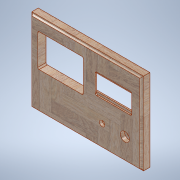
# Autodesk Inventor part: EW_Holzplatte
Saved by Autodesk Inventor 2020 (Build 240168000, 168)
## iProperties
Created: 2020-06-21
Part Number: EW_Holzplatte
Material: Eiche, Rot
Document SubType Name: Modeling
Designer: Johannes
Density: 0.673 g/cm^3
Appearance: Eiche - Fischgrätmuster
Author: Johannes
Autodesk Inventor part; units mm, degrees
ref_plane "YZ Plane" through (0, 0, 0) normal (1, 0, 0) x (0, 1, 0)
ref_plane "XZ Plane" through (0, 0, 0) normal (0, 1, 0) x (-1, 0, 0)
ref_plane "XY Plane" through (0, 0, 0) normal (0, 0, 1) x (1, 0, 0)
sketch "Skizze1" plane through (0, 0, 0) normal (0, 0, 1) x (1, 0, 0)
  line L0 (-122.5, 90) -> (122.5, 90)
  line L1 (122.5, 90) -> (122.5, -90)
  line L2 (122.5, -90) -> (-122.5, -90)
  line L3 (-122.5, -90) -> (-122.5, 90)
  line L4 (-122.5, 90) -> (122.5, -90) construction
  line L5 (122.5, 90) -> (-122.5, -90) construction
  point P0 (0, 0)
  dimension "d0" = 245
  dimension "d1" = 180
  constraints: 12 end point, 2 midpoint, 2 parallel, 1 horizontal, 1 perpendicular
  measures "d0" distance of L1.end L2.end
  measures "d1" distance of L0.end L1.end
extrude "Extrusion1" add sketch "Skizze1" along normal blind 18
sketch "Skizze3" plane through (0, 0, 18) normal (0, 0, 1) x (1, 0, 0)
  line L0 (20.5, 50.5) -> (100.5, 50.5)
  line L1 (100.5, 50.5) -> (100.5, 5.5)
  line L2 (100.5, 5.5) -> (20.5, 5.5)
  line L3 (20.5, 5.5) -> (20.5, 50.5)
  line L4 (20.5, 50.5) -> (100.5, 5.5) construction
  line L5 (100.5, 50.5) -> (20.5, 5.5) construction
  line L6 (122.5, 90) -> (-122.5, 90) projected
  line L7 (122.5, -90) -> (122.5, 90) projected
  point P0 (0, 0)
  point P1 (60.5, 28)
  dimension "d12" = 80
  dimension "d13" = 45
  dimension "d32" = 62
  dimension "d33" = 62
  constraints: 12 end point, 2 midpoint, 2 parallel, 1 horizontal, 1 perpendicular
  measures "d12" distance of L0.start L0.end
  measures "d13" distance of L2.end L0.start
  measures "d32" distance from line of L6 point (60.5, 28)
  measures "d33" distance from line of L7 point (60.5, 28)
extrude "Extrusion2" cut sketch "Skizze3" against normal blind 3
sketch "Skizze4" plane through (0, 0, 0) normal (0, 0, -1) x (-1, 0, 0)
  line L0 (-113, 69.75) -> (-8, 69.75)
  line L1 (-8, 69.75) -> (-8, -27.25)
  line L2 (-8, -27.25) -> (-113, -27.25)
  line L3 (-113, -27.25) -> (-113, 69.75)
  line L4 (-113, 69.75) -> (-8, -27.25) construction
  line L5 (-8, 69.75) -> (-113, -27.25) construction
  line L6 (-122.5, 90) -> (122.5, 90) projected
  line L7 (-122.5, -90) -> (-122.5, 90) projected
  point P0 (0, 0)
  point P1 (-60.5, 21.25)
  dimension "d20" = 62
  dimension "d21" = 105
  dimension "d22" = 97
  dimension "d23" = 20.25
  constraints: 12 end point, 2 midpoint, 2 parallel, 1 horizontal, 1 perpendicular
  measures "d20" distance from line of L7 point (-60.5, 21.25)
  measures "d21" distance of L0.start L0.end
  measures "d22" distance of L2.end L0.start
  measures "d23" distance between parallel lines of L0 L6
extrude "Extrusion3" cut sketch "Skizze4" against normal blind 6
sketch "Skizze5" plane through (0, 0, 6) normal (0, 0, -1) x (-1, 0, 0)
  line L0 (-113, 49) -> (-8, 49)
  line L1 (-8, 49) -> (-8, -6)
  line L2 (-8, -6) -> (-113, -6)
  line L3 (-113, -6) -> (-113, 49)
  line L4 (-113, 49) -> (-8, -6) construction
  line L5 (-8, 49) -> (-113, -6) construction
  line L6 (-122.5, 90) -> (122.5, 90) projected
  line L7 (-122.5, -90) -> (-122.5, 90) projected
  point P0 (0, 0)
  point P1 (-60.5, 21.5)
  dimension "d26" = 105
  dimension "d34" = 62
  dimension "d35" = 41
  dimension "d36" = 96
  constraints: 12 end point, 2 midpoint, 2 parallel, 1 horizontal, 1 perpendicular
  measures "d26" distance of L0.start L0.end
  measures "d34" distance from line of L7 point (-60.5, 21.5)
  measures "d35" distance between parallel lines of L6 L0
  measures "d36" distance between parallel lines of L2 L6
extrude "Extrusion4" cut sketch "Skizze5" against normal blind 6
sketch "Skizze14" plane through (0, 0, 12) normal (0, 0, -1) x (-1, 0, 0)
  line L0 (-113, 45.5) -> (-8, 45.5)
  line L1 (-8, 45.5) -> (-8, 10.5)
  line L2 (-8, 10.5) -> (-113, 10.5)
  line L3 (-113, 10.5) -> (-113, 45.5)
  line L4 (-113, 45.5) -> (-8, 10.5) construction
  line L5 (-8, 45.5) -> (-113, 10.5) construction
  line L6 (-122.5, -90) -> (-122.5, 90) projected
  line L7 (-122.5, 90) -> (122.5, 90) projected
  line L8 (-113, -27.25) -> (-113, 69.75) projected
  point P0 (0, 0)
  point P1 (-60.5, 28)
  dimension "d72" = 62
  dimension "d73" = 62
  dimension "d74" = 35
  constraints: 12 end point, 2 midpoint, 2 parallel, 1 collinear, 1 horizontal, 1 perpendicular
  measures "d72" distance from line of L6 point (-60.5, 28)
  measures "d73" distance from line of L7 point (-60.5, 28)
  measures "d74" distance of L2.end L0.start
extrude "Extrusion11" cut sketch "Skizze14" against normal blind 3
sketch "Skizze7" plane through (0, 0, 0) normal (0, 0, -1) x (-1, 0, 0)
  circle A0 centre (-35.5, -41.5) radius 6
  circle A1 centre (-85.5, -41.5) radius 3.5
  line L0 (-122.5, -90) -> (-122.5, 90) projected
  line L1 (-122.5, 90) -> (122.5, 90) projected
  point P0 (0, 0)
  dimension "d44" = 37
  dimension "d45" = 50
  dimension "d46" = 12
  dimension "d47" = 7
  dimension "d48" = 131.5
  constraints: 2 centre point, 1 horizontal alignment
  measures "d44" distance from line of L0 A1.centre
  measures "d45" distance of A0.centre A1.centre
  measures "d46" diameter of A0
  measures "d47" diameter of A1
  measures "d48" distance from line of L1 A0.centre
extrude "Extrusion6" cut sketch "Skizze7" against normal through all
sketch "Skizze8" plane through (0, 0, 0) normal (0, 0, -1) x (-1, 0, 0)
  line L0 (-43.5, -23.5) -> (-27.5, -23.5)
  line L1 (-27.5, -23.5) -> (-27.5, -59.5)
  line L2 (-27.5, -59.5) -> (-43.5, -59.5)
  line L3 (-43.5, -59.5) -> (-43.5, -23.5)
  line L4 (-43.5, -23.5) -> (-27.5, -59.5) construction
  line L5 (-27.5, -23.5) -> (-43.5, -59.5) construction
  circle A0 centre (-35.5, -41.5) radius 6 projected
  point P0 (0, 0)
  point P1 (-35.5, -41.5)
  dimension "d51" = 16
  dimension "d52" = 36
  constraints: 12 end point, 3 midpoint, 2 parallel, 1 coincident, 1 horizontal, 1 perpendicular
  measures "d51" distance of L0.start L0.end
  measures "d52" distance of L0.end L1.end
extrude "Extrusion7" cut sketch "Skizze8" against normal blind 12
sketch "Skizze9" plane through (0, 0, 0) normal (0, 0, -1) x (-1, 0, 0)
  line L0 (-91.5, -30.5) -> (-79.5, -30.5)
  line L1 (-79.5, -30.5) -> (-79.5, -52.5)
  line L2 (-79.5, -52.5) -> (-91.5, -52.5)
  line L3 (-91.5, -52.5) -> (-91.5, -30.5)
  circle A0 centre (-85.5, -41.5) radius 3.5 projected
  line L4 (-91.5, -30.5) -> (-79.5, -52.5) construction
  line L5 (-79.5, -30.5) -> (-91.5, -52.5) construction
  point P0 (0, 0)
  dimension "d55" = 12
  dimension "d56" = 22
  constraints: 12 end point, 2 midpoint, 2 parallel, 1 horizontal, 1 perpendicular
  measures "d55" distance of L1.end L2.end
  measures "d56" distance of L0.end L1.end
extrude "Extrusion8" cut sketch "Skizze9" against normal blind 5
sketch "Skizze10" plane through (0, 0, 18) normal (0, 0, 1) x (1, 0, 0)
  circle A0 centre (85.5, -41.5) radius 3.5 projected
  circle A1 centre (85.5, -41.5) radius 10
  point P0 (0, 0)
  dimension "d59" = 20
  constraints: 1 centre point, 1 coincident
  measures "d59" diameter of A1
extrude "Extrusion9" cut sketch "Skizze10" against normal blind 9
sketch "Skizze11" plane through (0, 0, 0) normal (0, 0, -1) x (-1, 0, 0)
  line L0 (5.5, 64) -> (105.5, 64)
  line L1 (105.5, 64) -> (105.5, -8)
  line L2 (105.5, -8) -> (5.5, -8)
  line L3 (5.5, -8) -> (5.5, 64)
  line L4 (5.5, 64) -> (105.5, -8) construction
  line L5 (105.5, 64) -> (5.5, -8) construction
  line L6 (-122.5, 90) -> (122.5, 90) projected
  line L7 (122.5, 90) -> (122.5, -90) projected
  point P0 (0, 0)
  point P1 (55.5, 28)
  dimension "d62" = 26
  dimension "d63" = 17
  dimension "d64" = 100
  dimension "d65" = 72
  constraints: 12 end point, 2 midpoint, 2 parallel, 1 horizontal, 1 perpendicular
  measures "d62" distance between parallel lines of L6 L0
  measures "d63" distance between parallel lines of L7 L1
  measures "d64" distance of L0.start L0.end
  measures "d65" distance of L0.end L1.end
extrude "Extrusion10" cut sketch "Skizze11" against normal through all
sketch "Skizze15" plane through (0, 0, 0) normal (0, 0, -1) x (-1, 0, 0)
  line L0 (105.5, -8) -> (5.5, -8) projected
  line L1 (5.5, -8) -> (-11, -8)
  line L2 (-11, -8) -> (-11, 49)
  line L3 (-11, 49) -> (5.5, 49)
  line L4 (5.5, 49) -> (5.5, -8)
  line L5 (-8, 69.75) -> (-8, -27.25) projected
  line L6 (-113, 49) -> (-8, 49) projected
  point P0 (0, 0)
  dimension "d80" = 3
  constraints: 8 end point, 2 parallel, 1 horizontal, 1 perpendicular, 1 point on line, 1 other
extrude "Extrusion12" cut sketch "Skizze15" against normal up to surface (12 mm away)
fillet "Rundung1" radius 3 32 edges at (20.5, 50.5, 16.5) (20.5, 5.5, 16.5) (100.5, 5.5, 16.5) (100.5, 50.5, 16.5) (113, 69.75, 3) (8, 69.75, 3) (8, -27.25, 3) (113, -27.25, 3) (113, 49, 9) (8, 49, 3) (113, -6, 9) (43.5, -27.25, 3) (27.5, -27.25, 3) (27.5, -23.5, 9) (43.5, -23.5, 9) (43.5, -59.5, 6) (27.5, -59.5, 6) (91.5, -30.5, 2.5) (79.5, -30.5, 2.5) (79.5, -52.5, 2.5) (91.5, -52.5, 2.5) (-5.5, 64, 9) (-5.5, -8, 15) (-105.5, -8, 9) (-105.5, 64, 9) (113, 45.5, 13.5) (113, 10.5, 13.5) (8, 45.5, 13.5) (8, 10.5, 13.5) (8, -8, 3) (-5.5, 49, 6) (11, -8, 9)
sketch "Skizze12" plane through (0, 0, 0) normal (1, 0, 0) x (0, 1, 0)
  circle A0 centre (90, 18) radius 4
  point P0 (0, 0)
  dimension "d69" = 8
  constraints: 1 centre point, 1 coincident
  measures "d69" diameter of A0
sketch "Skizze13" plane through (0, 0, 18) normal (0, 0, 1) x (1, 0, 0)
  line L0 (-122.5, 90) -> (-122.5, -90) projected
  line L1 (-122.5, -90) -> (122.5, -90) projected
  line L2 (122.5, -90) -> (122.5, 90) projected
  line L3 (122.5, 90) -> (-122.5, 90) projected
  line L4 (-102.5, 64) -> (-8.5, 64) projected
  arc A0 (-5.5, 61) -> (-8.5, 64) centre (-8.5, 61) ccw projected
  line L5 (-5.5, 61) -> (-5.5, -5) projected
  arc A1 (-8.5, -8) -> (-5.5, -5) centre (-8.5, -5) ccw projected
  line L6 (-8.5, -8) -> (-102.5, -8) projected
  arc A2 (-105.5, -5) -> (-102.5, -8) centre (-102.5, -5) ccw projected
  line L7 (-105.5, -5) -> (-105.5, 61) projected
  arc A3 (-102.5, 64) -> (-105.5, 61) centre (-102.5, 61) ccw projected
  circle A4 centre (85.5, -41.5) radius 10 projected
  circle A5 centre (35.5, -41.5) radius 6 projected
  line L8 (20.5, 8.5) -> (20.5, 47.5) projected
  arc A6 (23.5, 50.5) -> (20.5, 47.5) centre (23.5, 47.5) ccw projected
  line L9 (23.5, 50.5) -> (97.5, 50.5) projected
  arc A7 (100.5, 47.5) -> (97.5, 50.5) centre (97.5, 47.5) ccw projected
  line L10 (100.5, 47.5) -> (100.5, 8.5) projected
  arc A8 (97.5, 5.5) -> (100.5, 8.5) centre (97.5, 8.5) ccw projected
  line L11 (97.5, 5.5) -> (23.5, 5.5) projected
  arc A9 (20.5, 8.5) -> (23.5, 5.5) centre (23.5, 8.5) ccw projected
  point P0 (0, 0)
sweep "Sweeping1" cut profiles "Skizze12" path "Skizze13" path curves L1 L0 L3 L2
